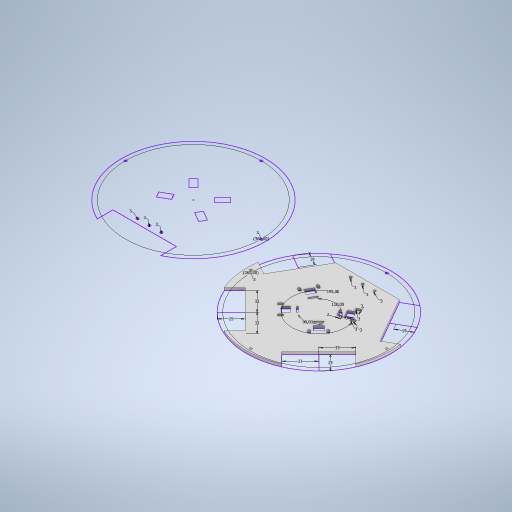
# Autodesk Inventor part: BaseV7.5
Saved by Autodesk Inventor 2024 (Build 280153000, 153)
## iProperties
Created: 2023-11-21
Part Number: BaseV7.5
Material: Generic
Document SubType Name: Modeling
Designer: felip
Density: 1 g/cm^3
Appearance: Default
Author: felip
Autodesk Inventor part; units mm, degrees
ref_plane "YZ Plane" through (0, 0, 0) normal (1, 0, 0) x (0, 1, 0)
ref_plane "XZ Plane" through (0, 0, 0) normal (0, 1, 0) x (-1, 0, 0)
ref_plane "XY Plane" through (0, 0, 0) normal (0, 0, 1) x (1, 0, 0)
sketch "Sketch1" plane through (0, 0, 0) normal (0, 1, 0) x (-1, 0, 0)
  circle A0 centre (0, 0) radius 90.0402
  line L0 (77.9423, -45) -> (56.2917, -32.5)
  line L1 (56.2917, -32.5) -> (39.7917, -61.0788)
  line L2 (39.7917, -61.0788) -> (56.0512, -70.4663)
  line L3 (56.2917, -32.5) -> (72.7917, -3.9212)
  line L4 (72.7917, -3.9212) -> (89.0512, -13.3086)
  line L5 (77.9423, -45) -> (61.4878, -35.5)
  line L6 (-77.9423, -45) -> (-56.2917, -32.5)
  line L7 (-56.2917, -32.5) -> (-72.7917, -3.9212)
  line L8 (-72.7917, -3.9212) -> (-89.0512, -13.3086)
  line L9 (-56.2917, -32.5) -> (-39.7917, -61.0788)
  line L10 (-39.7917, -61.0788) -> (-56.0512, -70.4663)
  line L11 (-77.9423, -45) -> (-61.4878, -35.5)
  line L12 (-24.1621, -13.95) -> (-28.4922, -16.45)
  line L13 (-24.1621, -13.95) -> (-21.564, -12.45)
  line L14 (-28.4922, -16.45) -> (-25.9922, -20.7801)
  line L15 (-28.4922, -16.45) -> (-30.9922, -12.1199)
  line L16 (-25.9922, -20.7801) -> (-30.9922, -12.1199)
  line L17 (-30.9922, -12.1199) -> (-24.064, -8.1199)
  line L18 (-24.064, -8.1199) -> (-19.064, -16.7801)
  line L19 (-19.064, -16.7801) -> (-25.9922, -20.7801)
  circle A1 centre (-34.9073, -10.3388) radius 1.5
  circle A2 centre (-26.4073, -25.0612) radius 1.5
  line L20 (-26.4073, -25.0612) -> (-23.8092, -23.5612)
  line L21 (-34.9073, -10.3388) -> (-32.3092, -8.8388)
  circle A3 centre (-32.3092, -8.8388) radius 1.5
  circle A4 centre (-23.8092, -23.5612) radius 1.5
  line L22 (-23.0592, -24.8603) -> (-25.6573, -26.3603)
  line L23 (-24.5592, -22.2622) -> (-27.1573, -23.7622)
  line L24 (-31.5592, -10.1378) -> (-34.1573, -11.6378)
  line L25 (-35.6573, -9.0397) -> (-33.0592, -7.5397)
  line L26 (-16.3679, -9.45) -> (-18.8679, -5.1199)
  line L27 (-16.3679, -9.45) -> (-13.8679, -13.7801)
  line L28 (-13.8679, -13.7801) -> (-18.8679, -5.1199) construction
  line L29 (-13.5019, -12.4141) -> (-17.5019, -5.4859)
  line L30 (-19.2339, -6.4859) -> (-15.2339, -13.4141)
  arc A5 (-15.2339, -13.4141) -> (-13.5019, -12.4141) centre (-14.3679, -12.9141) ccw
  arc A6 (-17.5019, -5.4859) -> (-19.2339, -6.4859) centre (-18.3679, -5.9859) ccw
  line L31 (39.7917, -61.0788) -> (-39.7917, -61.0788)
  line L32 (15.2339, -13.4141) -> (19.2339, -6.4859)
  arc A7 (19.2339, -6.4859) -> (17.5019, -5.4859) centre (18.3679, -5.9859) ccw
  line L33 (17.5019, -5.4859) -> (13.5019, -12.4141)
  arc A8 (13.5019, -12.4141) -> (15.2339, -13.4141) centre (14.3679, -12.9141) ccw
  line L34 (19.064, -16.7801) -> (24.064, -8.1199)
  line L35 (25.9922, -20.7801) -> (19.064, -16.7801)
  line L36 (30.9922, -12.1199) -> (25.9922, -20.7801)
  line L37 (24.064, -8.1199) -> (30.9922, -12.1199)
  circle A9 centre (23.8092, -23.5612) radius 1.5
  line L38 (24.5592, -22.2622) -> (27.1573, -23.7622)
  circle A10 centre (26.4073, -25.0612) radius 1.5
  line L39 (25.6573, -26.3603) -> (23.0592, -24.8603)
  line L40 (31.5592, -10.1378) -> (34.1573, -11.6378)
  circle A11 centre (32.3092, -8.8388) radius 1.5
  line L41 (33.0592, -7.5397) -> (35.6573, -9.0397)
  circle A12 centre (34.9073, -10.3388) radius 1.5
  line L42 (31.042, 19.0212) -> (28.9207, 16.8999)
  circle A13 centre (28.9207, 16.8999) radius 1.5
  line L43 (27.86, 17.9605) -> (29.9813, 20.0818)
  line L44 (32.1026, 17.9605) -> (29.9813, 15.8392)
  circle A14 centre (31.042, 19.0212) radius 1.5
  line L45 (26.7993, 19.7283) -> (21.1425, 14.0714)
  line L46 (19.7283, 26.7993) -> (26.7993, 19.7283)
  line L47 (14.0714, 21.1425) -> (19.7283, 26.7993)
  line L48 (21.1425, 14.0714) -> (14.0714, 21.1425)
  line L49 (16.8999, 11.243) -> (11.243, 16.8999)
  arc A15 (11.243, 16.8999) -> (9.8288, 15.4856) centre (10.5359, 16.1927) ccw
  line L50 (9.8288, 15.4856) -> (15.4856, 9.8288)
  arc A16 (15.4856, 9.8288) -> (16.8999, 11.243) centre (16.1927, 10.5359) ccw
  line L51 (17.9605, 27.86) -> (20.0818, 29.9813)
  circle A17 centre (16.8999, 28.9207) radius 1.5
  line L52 (15.8392, 29.9813) -> (17.9605, 32.1026)
  circle A18 centre (19.0212, 31.042) radius 1.5
  line L53 (-15.4856, 9.8288) -> (-9.8288, 15.4856)
  arc A19 (-9.8288, 15.4856) -> (-11.243, 16.8999) centre (-10.5359, 16.1927) ccw
  line L54 (-11.243, 16.8999) -> (-16.8999, 11.243)
  arc A20 (-16.8999, 11.243) -> (-15.4856, 9.8288) centre (-16.1927, 10.5359) ccw
  circle A21 centre (-28.9207, 16.8999) radius 1.5
  circle A22 centre (-31.042, 19.0212) radius 1.5
  line L55 (-29.9813, 15.8392) -> (-32.1026, 17.9605)
  line L56 (-27.86, 17.9605) -> (-29.9813, 20.0818)
  line L57 (-21.1425, 14.0714) -> (-26.7993, 19.7283)
  line L58 (-26.7993, 19.7283) -> (-19.7283, 26.7993)
  line L59 (-19.7283, 26.7993) -> (-14.0714, 21.1425)
  line L60 (-14.0714, 21.1425) -> (-21.1425, 14.0714)
  circle A23 centre (-16.8999, 28.9207) radius 1.5
  line L61 (-17.9605, 32.1026) -> (-15.8392, 29.9813)
  circle A24 centre (-19.0212, 31.042) radius 1.5
  line L62 (-17.9605, 27.86) -> (-20.0818, 29.9813)
  line L63 (63.6396, 63.6396) -> (45.9619, 45.9619)
  line L64 (45.9619, 45.9619) -> (22.6274, 69.2965)
  line L65 (22.6274, 69.2965) -> (35.9033, 82.5724)
  line L66 (45.9619, 45.9619) -> (69.2965, 22.6274)
  line L67 (69.2965, 22.6274) -> (82.5724, 35.9033)
  line L68 (-63.6396, 63.6396) -> (-45.9619, 45.9619)
  line L69 (-45.9619, 45.9619) -> (-69.2965, 22.6274)
  line L70 (-69.2965, 22.6274) -> (-82.5724, 35.9033)
  line L71 (-45.9619, 45.9619) -> (-22.6274, 69.2965)
  line L72 (-22.6274, 69.2965) -> (-35.9033, 82.5724)
  circle A25 centre (85, 0) radius 1.5
  circle A26 centre (0, 85) radius 1.5
  circle A27 centre (-85, 0) radius 1.5
  circle A28 centre (0, -85) radius 1.5
  circle A29 centre (15, -55.0788) radius 1.5
  circle A30 centre (0, -55.0788) radius 1.5
  circle A31 centre (-15, -55.0788) radius 1.5
  point P0 (-16.3679, -9.45)
  point P1 (16.8999, 9.8288)
  dimension "d12" = 19
  dimension "d18" = 19
  dimension "d20" = 5
  dimension "d21" = 3
  dimension "d27" = 3
  dimension "d28" = 3
  dimension "d29" = 3
  dimension "d30" = 3
  dimension "d31" = 6
  dimension "d32" = 5
  dimension "d33" = 5
  dimension "d34" = 2
  dimension "d37" = 120
  dimension "d41" = 195
  dimension "d45" = 90
  dimension "d47" = 25
  dimension "d48" = 33
  dimension "d49" = 33
  dimension "d50" = 25
  dimension "d51" = 33
  dimension "d52" = 33
  dimension "d54" = 3
  dimension "d57" = 360
  dimension "d64" = 3
  dimension "d65" = 3
  dimension "d66" = 3
  constraints: 148 end point, 51 point on circle, 31 centre point, 13 perpendicular, 6 tangent, 4 coincident, 4 parallel, 4 point on line, 1 horizontal, 1 midpoint, 139 other
  measures "d12" distance of L0.start L5.end
  measures "d18" distance of L6.start L11.end
  measures "d20" distance of L12.start L12.end
  measures "d21" distance of L12.start L13.end
  measures "d27" diameter of A1
  measures "d28" diameter of A2
  measures "d29" diameter of A3
  measures "d30" diameter of A4
  measures "d31" distance of L13.end L26.start
  measures "d32" distance of L26.start L26.end
  measures "d33" distance of L26.start L27.end
  measures "d34" diameter of A6
  measures "d47" distance of L63.start L63.end
  measures "d48" distance of L63.end L64.end
  measures "d49" distance of L63.end L66.end
  measures "d50" distance of L68.start L68.end
  measures "d51" distance of L68.end L69.end
  measures "d52" distance of L68.end L71.end
  measures "d54" diameter of A25
  measures "d64" diameter of A29
  measures "d65" diameter of A30
  measures "d66" diameter of A31
extrude "Extrusion2" add sketch "Sketch1" along normal blind 3 contours A0 L4 L3 L1 L31 L9 L7 L8 L70 L69 L71 L72 L65 L64 L66 L67
sketch "Sketch2" plane through (0, 3, 0) normal (0, 1, 0) x (1, 0, 0)
  arc A0 (-157.438, -40.5996) -> (-237.0213, -40.5996) centre (-197.2297, 40.1708) ccw
  line L0 (-225.7219, 23.7208) -> (-223.7219, 20.2567)
  line L1 (-225.7219, 23.7208) -> (-227.7219, 27.1849)
  line L2 (-213.5976, 30.7208) -> (-215.5976, 34.1849)
  line L3 (-213.5976, 30.7208) -> (-211.5976, 27.2567)
  line L4 (-157.438, -20.908) -> (-237.0213, -20.908)
  circle A1 centre (-112.2297, 40.1708) radius 1.5
  circle A2 centre (-197.2297, 125.1708) radius 1.5
  circle A3 centre (-282.2297, 40.1708) radius 1.5
  circle A4 centre (-197.2297, -44.8292) radius 1.5
  circle A5 centre (-182.2297, -14.908) radius 1.5
  circle A6 centre (-197.2297, -14.908) radius 1.5
  circle A7 centre (-212.2297, -14.908) radius 1.5
  line L5 (-215.5976, 34.1849) -> (-211.5976, 27.2567)
  line L6 (-211.5976, 27.2567) -> (-223.7219, 20.2567)
  line L7 (-223.7219, 20.2567) -> (-227.7219, 27.1849)
  line L8 (-227.7219, 27.1849) -> (-215.5976, 34.1849)
  line L9 (-213.4224, 50.7067) -> (-207.7656, 56.3636)
  line L10 (-207.7656, 56.3636) -> (-217.6651, 66.2631)
  line L11 (-217.6651, 66.2631) -> (-223.3219, 60.6062)
  line L12 (-223.3219, 60.6062) -> (-213.4224, 50.7067)
  line L13 (-186.6938, 56.3636) -> (-181.0369, 50.7067)
  line L14 (-181.0369, 50.7067) -> (-171.1374, 60.6062)
  line L15 (-171.1374, 60.6062) -> (-176.7943, 66.2631)
  line L16 (-176.7943, 66.2631) -> (-186.6938, 56.3636)
  line L17 (-178.8618, 34.1849) -> (-182.8618, 27.2567)
  line L18 (-182.8618, 27.2567) -> (-170.7374, 20.2567)
  line L19 (-170.7374, 20.2567) -> (-166.7374, 27.1849)
  line L20 (-166.7374, 27.1849) -> (-178.8618, 34.1849)
  line L21 (-223.7219, 20.2567) -> (-227.7219, 27.1849)
  line L22 (-219.9278, 109.3966) -> (-219.8571, 109.4673)
  line L23 (-237.0213, -20.908) -> (-237.0213, -40.5996)
  line L24 (-157.438, -20.908) -> (-157.438, -40.5996)
  point P0 (0, 0)
  point P1 (-213.5976, 30.7208)
  dimension "d98" = 3
  dimension "d99" = 360
  dimension "d100" = 3
  dimension "d101" = 3
  dimension "d102" = 3
  constraints: 50 end point, 9 parallel, 8 centre point, 4 perpendicular, 2 point on circle, 1 coincident, 1 horizontal, 1 point on line, 1 vertical, 9 other
  measures "d98" diameter of A1
  measures "d100" diameter of A5
  measures "d101" diameter of A6
  measures "d102" diameter of A7
body "Solid2"
